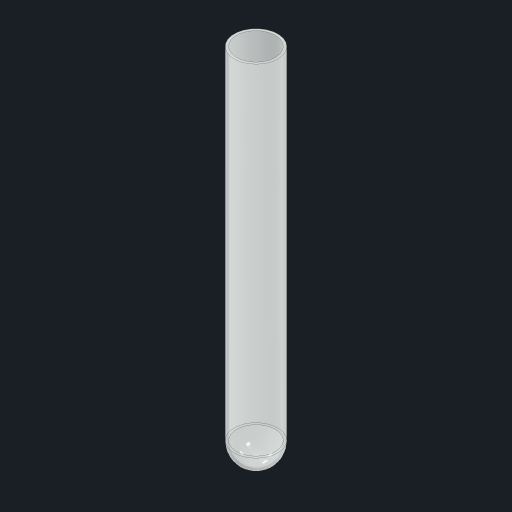
# Autodesk Inventor part: Test Tube
Saved by Autodesk Inventor 2023.1 (Build 271208000, 208)
## iProperties
Created: 2022-11-01
Part Number: Test Tube
Material: Glass
Document SubType Name: Modeling
Designer: Jarrett
Density: 2.18 g/cm^3
Appearance: Clear
Author: Jarrett
Autodesk Inventor part; units mm, degrees
ref_plane "YZ Plane" through (0, 0, 0) normal (1, 0, 0) x (0, 1, 0)
ref_plane "XZ Plane" through (0, 0, 0) normal (0, 1, 0) x (-1, 0, 0)
ref_plane "XY Plane" through (0, 0, 0) normal (0, 0, 1) x (1, 0, 0)
sketch "Sketch1" plane through (0, 0, 0) normal (0, 0, 1) x (1, 0, 0)
  arc A0 (0, 0) -> (9, 9) centre (0, 9) ccw
  line L0 (9, 9) -> (9, 150)
  line L1 (9, 150) -> (8, 150)
  line L2 (8, 150) -> (8, 9)
  arc A1 (0, 1) -> (8, 9) centre (0, 9) ccw
  line L3 (0, -32.2368) -> (0, 180.3728) projected
  line L4 (0, 1) -> (0, 0)
  point P0 (0, 0)
  dimension "d0" = 18
  dimension "d1" = 1
  dimension "d2" = 150
  constraints: 8 end point, 5 point on circle, 3 point on line, 2 centre point, 2 perpendicular, 2 tangent, 2 vertical, 1 coincident
  measures "d0" diameter of L0 L3
  measures "d1" distance between parallel lines of L0 L2
  measures "d2" distance from line of point (0, 0) L1
revolve "Revolution1" add sketch "Sketch1" angle 360 about axis through (0, -10, 0) along (0, 1, 0)
body "Solid1"
